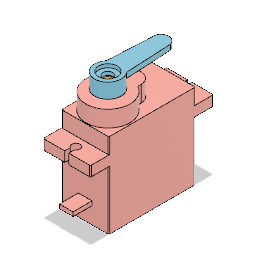
Servo SG90 (Autodesk Fusion 360 design; units mm, degrees)
Autodesk Fusion 360 part; units mm, degrees
note: some values were not read from the file. Chosen so that the rebuilt part matches the saved one: which face or edge a step refers to.
sketch "Body" plane through (0, 0, 0) normal (0, 1, 0) x (1, 0, 0) in component "servo"
  line L0 (6.25, -11.375) -> (-6.25, -11.375)
  line L1 (-6.25, -11.375) -> (-6.25, 11.375)
  line L2 (-6.25, 11.375) -> (6.25, 11.375)
  line L3 (6.25, 11.375) -> (6.25, -11.375)
  line L4 (6.25, -11.375) -> (-6.25, 11.375) construction
  line L5 (-6.25, -11.375) -> (6.25, 11.375) construction
  dimension "d6" = 12.5
  dimension "d7" = 22.75
  dimension "d52" = 0
  dimension "d53" = 0
  dimension "d54" = 0
  dimension "d55" = 0
extrude "Extrude1" add sketch "Body" along normal blind 22.35 makes body 1 in component "servo"
sketch "Tab" plane through (0, 0, 11.375) normal (0, 0, 1) x (1, 0, 0) in component "servo"
  line L0 (-6.25, 0) -> (6.25, 0)
  line L1 (6.25, 0) -> (6.25, 22.35)
  line L2 (6.25, 22.35) -> (-6.25, 22.35)
  line L3 (-6.25, 22.35) -> (-6.25, 0)
  line L4 (-6.25, 18.2) -> (6.25, 18.2)
  line L5 (6.25, 18.2) -> (6.25, 15.55)
  line L6 (6.25, 15.55) -> (-6.25, 15.55)
  line L7 (-6.25, 15.55) -> (-6.25, 18.2)
  dimension "d10" = 4.15
  dimension "d11" = 2.65
extrude "Extrude2" add sketch "Tab" along normal blind 4.85 contours L1 L3 L4 L5 L6 L7 bodies 1 in component "servo"
hole "Hole1" at (0, 18.2, 13.8) direction (0, -1, 0) diameter 2.2 depth 2.65 tip angle 118 bodies 1 in component "servo"
fillet "Fillet1" radius 0.25 2 edges at (6.25, 16.875, 16.225) (-6.25, 16.875, 16.225) on bodies 1 in component "servo"
sketch "Notch" plane through (0, 0, 16.225) normal (0, 0, 1) x (1, 0, 0) in component "servo"
  line L0 (-6, 18.2) -> (-6, 15.55)
  line L1 (-6, 15.55) -> (6, 15.55)
  line L2 (6, 15.55) -> (6, 18.2)
  line L3 (6, 18.2) -> (-6, 18.2)
  line L4 (-0.525, 18.2) -> (0.525, 18.2)
  line L5 (0.525, 18.2) -> (0.525, 15.55)
  line L6 (0.525, 15.55) -> (-0.525, 15.55)
  line L7 (-0.525, 15.55) -> (-0.525, 18.2)
  dimension "d20" = 1.05
extrude "Extrude3" cut sketch "Notch" along normal up to surface contours L1 L3 L4 L5 L6 L7 end surface at (0.0548, 17.3167, 14.8986) on bodies 1 bodies 1 in component "servo"
mirror "Mirror1" about plane through (0, 0, 0) normal (0, 0, 1) of "Extrude2", "Hole1", "Fillet1", "Extrude3" in component "servo"
sketch "Bump" plane through (0, 22.35, 0) normal (0, 1, 0) x (-1, 0, 0) in component "servo"
  line L0 (-6.25, -11.375) -> (6.25, -11.375)
  line L1 (6.25, -11.375) -> (6.25, 11.375)
  line L2 (6.25, 11.375) -> (-6.25, 11.375)
  line L3 (-6.25, 11.375) -> (-6.25, -11.375)
  line L4 (-2.8, -0.625) -> (-2.8, 0.2671)
  line L5 (2.8, 0.2671) -> (2.8, -0.625)
  arc A0 (-2.8, -0.625) -> (2.8, -0.625) centre (0, -0.625) ccw
  arc A1 (2.8, 0.2671) -> (-2.8, 0.2671) centre (0, 5.375) ccw
  dimension "d23" = 11.65
  dimension "d24" = 6
  dimension "d25" = 5.6
  dimension "d26" = 6
  dimension "d27" = 6.25
  dimension "d28" = 6.25
  measures "d23" diameter of A1
  measures "d24" distance of L2
  measures "d25" diameter of A0
  measures "d26" distance of origin
  measures "d27" distance of L3
  measures "d28" distance of L3 origin
extrude "Extrude4" add sketch "Bump" along normal blind 4.3 contours L4 L5 A0 A1 bodies 1 in component "servo"
fillet "Fillet2" radius 0.25 8 edges at (6.25, 7.775, 11.375) (6.25, 20.275, 11.375) (-6.25, 20.275, 11.375) (-6.25, 7.775, 11.375) (6.25, 7.775, -11.375) (6.25, 20.275, -11.375) (-6.25, 20.275, -11.375) (-6.25, 7.775, -11.375) on bodies 1 in component "servo"
sketch "Wire" plane through (0, 0, 11.375) normal (0, 0, 1) x (1, 0, 0) in component "servo"
  line L0 (-6, 15.55) -> (-6, 0)
  line L1 (-6, 0) -> (6, 0)
  line L2 (6, 0) -> (6, 15.55)
  line L3 (6, 15.55) -> (-6, 15.55)
  line L4 (-1.8, 5.5) -> (1.8, 5.5)
  line L5 (1.8, 5.5) -> (1.8, 4.4)
  line L6 (1.8, 4.4) -> (-1.8, 4.4)
  line L7 (-1.8, 4.4) -> (-1.8, 5.5)
  dimension "d32" = 1.1
  dimension "d33" = 3.6
  dimension "d34" = 5.5
  measures "d34" distance of L1
extrude "Extrude5" add sketch "Wire" along normal blind 5 contours L4 L5 L6 L7 bodies 1 in component "servo"
hole "Hole2" at (0, 26.65, 5.375) direction (0, -1, 0) diameter 4.92 depth 15 tip angle 180 bodies 1 in component "servo"
cylinder "CylinderPrimitive1" add diameter 4.92 height 2.72 placed x (1, 0, 0) y (0, 0, -1) z (0, 1, 0) at (0, 26.65, 5.375) separate body makes body 2 in component "splined-drive"
extrude "Extrude1'" add 1 faces at (-0.4548, 26.65, 5.9711) along direction (0, -1, 0) blind 15 on bodies 2 bodies 2 in component "splined-drive"
hole "Hole1'" at (0, 29.37, 5.375) direction (0, -1, 0) diameter 1.95 depth 5 tip angle 180 bodies 2 in component "splined-drive"
chamfer "Chamfer1" distance 0.25 angle 45 1 edges at (-2.2935, 29.37, 6.2646) on bodies 2 in component "splined-drive"
sketch "Sketch1" plane through (0, 29.37, 0) normal (0, 1, 0) x (-1, 0, 0) in component "horn"
  circle A0 centre (0, 5.375) radius 3.5
  circle A1 centre (0, 5.375) radius 2.46
  circle A2 centre (0, 5.375) radius 1.31
extrude "Extrude3'" add sketch "Sketch1" against normal blind 2.08 separate body contours A0 makes body 3 in component "horn"
extrude "Extrude6" add 1 faces at (-3.1311, 29.37, 5.0789) along direction (0, 1, 0) blind 1.83 on bodies 3 bodies 3 in component "horn"
extrude "Extrude4'" add sketch "Sketch1" along normal blind 0.9 contours A1 bodies 3 in component "horn"
sketch "Sketch4" plane through (0, 31.2, 0) normal (0, 1, 0) x (-1, 0, 0) in component "horn"
  circle A0 centre (0, 5.375) radius 2.46
  circle A1 centre (0, 5.375) radius 3.5
  line L0 (2.67, 3.112) -> (2.04, -9.105)
  line L1 (-2.67, 3.112) -> (-2.04, -9.105)
  arc A2 (-2.04, -9.105) -> (2.04, -9.105) centre (0, -8.6045) ccw
extrude "Extrude7" add sketch "Sketch4" against normal blind 1.41 contours A1 L0 L1 A2 bodies 3 in component "horn"
component "servo" placed x (1, 0, 0) y (0, 1, 0) z (0, 0, 1) at (0, 0, 0)
component "splined-drive" placed x (1, 0, 0) y (0, 1, 0) z (0, 0, 1) at (0, 0, 0)
component "horn" placed x (1, 0, 0) y (0, 1, 0) z (0, 0, 1) at (0, 0, 0)
